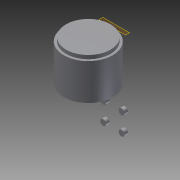
# Autodesk Inventor part: Grounded banana jack
Saved by Autodesk Inventor 2012 (Build 160160000, 160)
## iProperties
Created: 2017-04-26
Part Number: Grounded banana jack
Material: Default
Document SubType Name: Modeling
Designer: Brandon
Density: 1 g/cm^3
Author: Brandon
Autodesk Inventor part; units mm, degrees
ref_plane "YZ Plane" through (0, 0, 0) normal (1, 0, 0) x (0, 1, 0)
ref_plane "XY Plane" through (0, 0, 0) normal (0, 0, 1) x (1, 0, 0)
sketch "Sketch1" plane through (0, 0, 0) normal (0, 0, 1) x (1, 0, 0)
  circle A0 centre (-2.54, 2.54) radius 0.8001
  circle A1 centre (2.54, 2.54) radius 0.8001
  circle A2 centre (-2.54, -2.54) radius 0.8001
  circle A3 centre (2.54, -2.54) radius 0.8001
  point P0 (0, 0)
  dimension "d0" = 1.6002
  dimension "d1" = 1.6002
  dimension "d2" = 1.6002
  dimension "d3" = 1.6002
  dimension "d4" = 5.08
  dimension "d5" = 5.08
  dimension "d6" = 5.08
  dimension "d7" = 2.54
  dimension "d8" = 2.54
  constraints: 4 centre point
  measures "d0" diameter of A0
  measures "d1" diameter of A1
  measures "d2" diameter of A2
  measures "d3" diameter of A3
  measures "d4" distance of A1.centre A0.centre
  measures "d5" distance of A0.centre A2.centre
  measures "d6" distance of A2.centre A3.centre
  measures "d7" horizontal distance of point (0, 0) A0.centre
  measures "d8" horizontal distance of point (0, 0) A0.centre
extrude "Extrusion1" add sketch "Sketch1" along normal blind 1
ref_plane "Work Plane1" through (0, 21.4376, 0) normal (0, 1, 0) x (-1, 0, 0)
sketch "Sketch2" plane through (0, 21.4376, 0) normal (0, 1, 0) x (-1, 0, 0)
  circle A0 centre (0, 7.62) radius 6.096
  circle A1 centre (0, 7.62) radius 6.731
  point P0 (0, 0)
  dimension "d12" = 12.192
  dimension "d13" = 13.462
  dimension "d14" = 7.62
  constraints: 2 centre point, 1 coincident
  measures "d12" diameter of A0
  measures "d13" diameter of A1
  measures "d14" distance of point (0, 0) A1.centre
extrude "Extrusion2" add sketch "Sketch2" along normal blind 1 contours A0
extrude "Extrusion3" add sketch "Sketch2" against normal blind 10 contours A0 | A1
body "Solid1"
